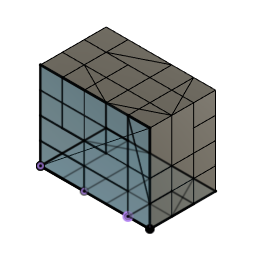
Aula2 v5 (Autodesk Fusion 360 design; units mm, degrees)
Autodesk Fusion 360 part; units mm, degrees
sketch "FRENTE" plane through (0, 0, 0) normal (0, 1, 0) x (1, 0, 0) in component "exercicio1"
  line L0 (0, 0) -> (50, 0)
  line L1 (50, 0) -> (50, -40)
  line L2 (50, -40) -> (0, -40)
  line L3 (0, -40) -> (0, 0)
  line L4 (0, 0) -> (20, 0)
  line L5 (20, 0) -> (20, -10)
  line L6 (20, -10) -> (0, -10)
  line L7 (0, -10) -> (0, 0)
  line L8 (0, -40) -> (30, -40)
  line L9 (30, -40) -> (30, -20)
  line L10 (30, -20) -> (0, -20)
  line L11 (0, -20) -> (0, -40)
  line L12 (50, -40) -> (40, -40)
  line L13 (40, -40) -> (40, 0)
  line L14 (40, 0) -> (50, 0)
  line L15 (50, 0) -> (50, -40)
  dimension "d1" = 50
  dimension "d2" = 40
  dimension "d3" = 10
  dimension "d4" = 10
  dimension "d5" = 20
  dimension "d6" = 20
  dimension "d7" = 30
  constraint horizontal L0
  constraint vertical L1
  constraint horizontal L2
  constraint vertical L3
  constraint coincident L0.start L3.end
  constraint horizontal L4
  constraint vertical L5
  constraint horizontal L6
  constraint vertical L7
  constraint horizontal L8
  constraint vertical L9
  constraint horizontal L10
  constraint vertical L11
  constraint horizontal L12
  constraint vertical L13
  constraint horizontal L14
  constraint vertical L15
  constraint coincident L0 L13.end
  measures "d1" distance of L1.end L2.end
  measures "d2" distance of L0.end L1.end
  measures "d3" distance of L1 L13
  measures "d4" distance of L4.end L5.end
  measures "d5" distance of L5.end L6.end
  measures "d6" distance of L8.end L9.end
  measures "d7" distance of L9.end L10.end
sketch "TOPO" plane through (0, 0, 0) normal (0, 0, 1) x (1, 0, 0) in component "exercicio1"
  line L0 (0, 0) -> (50, 0)
  line L1 (50, 0) -> (50, 30)
  line L2 (50, 30) -> (0, 30)
  line L3 (0, 30) -> (0, 0)
  line L4 (40, 10) -> (50, 10)
  line L5 (50, 10) -> (50, 20)
  line L6 (50, 20) -> (40, 20)
  line L7 (40, 20) -> (40, 10)
  line L8 (0, 0) -> (20, 0)
  line L9 (20, 0) -> (20, 20)
  line L10 (20, 20) -> (0, 20)
  line L11 (0, 20) -> (0, 0)
  point P0 (50, 0)
  point P1 (40, 0)
  point P2 (40, 0)
  point P3 (20, 0)
  dimension "d15" = 30
  constraint horizontal L0
  constraint vertical L1
  constraint horizontal L2
  constraint vertical L3
  constraint coincident L0.start L3.end
  constraint coincident P0 L0.end
  constraint horizontal L4
  constraint vertical L5
  constraint horizontal L6
  constraint vertical L7
  constraint midpoint L1 L5
  constraint coincident L7 P2
  constraint equal L4 L7
  constraint horizontal L8
  constraint vertical L9
  constraint horizontal L10
  constraint vertical L11
  constraint coincident L9 P3
  constraint equal L9 L10
  measures "d15" distance of P0 L1.end
extrude "Extrude1" add sketch "FRENTE" along normal up to surface (30 mm away) contours L0 L3 L4 L5 L6 L7 | L0 L2 L3 L5 L6 L9 L10 L13 | L0 L1 L2 L12 L13 L14 L15 makes body 1 in component "exercicio1"
extrude "Extrude3" cut sketch "TOPO" along normal up to surface (10 mm away) contours L0 L3 L8 L9 L10 L11 bodies 1 in component "exercicio1"
extrude "Extrude4" cut sketch "FRENTE" along normal up to surface (10 mm away) from surface at 10 contours L0 L1 L2 L12 L13 L14 L15 bodies 1 in component "exercicio1"
sketch "Sketch1" plane through (0, 0, 0) normal (0, 1, 0) x (1, 0, 0) in component "Exercicio2"
  line L0 (0, 0) -> (50, 0)
  line L1 (50, 0) -> (50, -40)
  line L2 (50, -40) -> (0, -40)
  line L3 (0, -40) -> (0, 0)
  line L4 (10, -40) -> (30, -40)
  line L5 (30, -40) -> (30, -20)
  line L6 (30, -20) -> (10, -20)
  line L7 (10, -20) -> (10, -40)
  line L8 (40, -40) -> (50, -10)
  dimension "d25" = 40
  dimension "d26" = 20
  dimension "d27" = 20
  dimension "d28" = 50
  dimension "d29" = 10
  dimension "d30" = 10
  dimension "d32" = 10
  constraint horizontal L0
  constraint vertical L1
  constraint horizontal L2
  constraint vertical L3
  constraint coincident L0.start L3.end
  constraint horizontal L4
  constraint vertical L5
  constraint horizontal L6
  constraint vertical L7
  constraint coincident L2 L4.start
  constraint coincident L2 L8.start
  constraint coincident L1 L8.end
  measures "d25" distance of L0.start L2.end
  measures "d26" distance of L5.end L6.end
  measures "d27" distance of L4.end L5.end
  measures "d28" distance of L0.start L0.end
  measures "d29" distance of L0.end L8.end
  measures "d30" distance of L1.end L8.start
  measures "d32" distance of L3 L7
sketch "Sketch2" plane through (0, 0, 0) normal (0, 0, 1) x (1, 0, 0) in component "Exercicio2"
  line L0 (0, 0) -> (50, 0)
  line L1 (50, 0) -> (50, 30)
  line L2 (50, 30) -> (0, 30)
  line L3 (0, 30) -> (0, 0)
  line L4 (0, 0) -> (10, 0)
  line L5 (10, 0) -> (10, 30)
  line L6 (10, 30) -> (0, 30)
  line L7 (0, 30) -> (0, 0)
  line L8 (30, 0) -> (50, 0)
  line L9 (50, 0) -> (50, 30)
  line L10 (50, 30) -> (30, 30)
  line L11 (30, 30) -> (30, 0)
  line L12 (50, 0) -> (40, 0)
  line L13 (40, 0) -> (40, 20)
  line L14 (40, 20) -> (50, 20)
  line L15 (50, 20) -> (50, 0)
  point P0 (50, 0)
  dimension "d33" = 30
  dimension "d34" = 10
  dimension "d35" = 10
  dimension "d36" = 10
  dimension "d37" = 10
  constraint horizontal L0
  constraint vertical L1
  constraint horizontal L2
  constraint vertical L3
  constraint coincident L0.start L3.end
  constraint horizontal L4
  constraint vertical L5
  constraint horizontal L6
  constraint vertical L7
  constraint coincident L2 L5.end
  constraint horizontal L8
  constraint vertical L9
  constraint horizontal L10
  constraint vertical L11
  constraint coincident L0 L8.start
  constraint horizontal L12
  constraint vertical L13
  constraint horizontal L14
  constraint vertical L15
  constraint coincident L15 P0
  measures "d33" distance of L1.end P0
  measures "d34" distance of L10 L14
  measures "d35" distance of L11 L13
  measures "d36" distance of L3 L5
  measures "d37" distance of L1 L13
extrude "Extrude1'" add sketch "Sketch1" along normal up to surface (30 mm away) separate body contours L0 L1 L2 L3 L5 L6 L7 L8 | L1 L2 L8 makes body 2 in component "Exercicio2"
extrude "Extrude2" cut sketch "Sketch1" along normal up to surface (20 mm away) contours L1 L2 L8 bodies 2 in component "Exercicio2"
sketch "Sketch1 (2)" plane through (0, 0, 0) normal (0, 1, 0) x (1, 0, 0) in component "Exercicio3"
  line L0 (0, 0) -> (50, 0)
  line L1 (50, 0) -> (50, -40)
  line L2 (50, -40) -> (0, -40)
  line L3 (0, -40) -> (0, 0)
  line L4 (10, -40) -> (30, -40)
  line L5 (30, -40) -> (30, -20)
  line L6 (30, -20) -> (10, -20)
  line L7 (10, -20) -> (10, -40)
  line L8 (40, -40) -> (50, -10)
  dimension "d42" = 40
  dimension "d43" = 50
  dimension "d44" = 10
  dimension "d45" = 10
  dimension "d46" = 20
  dimension "d48" = 10
  constraint horizontal L0
  constraint vertical L1
  constraint horizontal L2
  constraint vertical L3
  constraint coincident L0.start L3.end
  constraint horizontal L4
  constraint vertical L5
  constraint horizontal L6
  constraint vertical L7
  constraint coincident L2 L4.start
  constraint coincident L2 L8.start
  constraint coincident L1 L8.end
  constraint equal L5 L6
  measures "d42" distance of L0.start L2.end
  measures "d43" distance of L0.start L0.end
  measures "d44" distance of L0.end L8.end
  measures "d45" distance of L1.end L8.start
  measures "d46" distance of L5.end L6.end
  measures "d48" distance of L3 L7
sketch "Sketch2 (2)" plane through (0, 0, 0) normal (0, 0, 1) x (1, 0, 0) in component "Exercicio3"
  line L0 (0, 0) -> (50, 0)
  line L1 (50, 0) -> (50, 30)
  line L2 (50, 30) -> (0, 30)
  line L3 (0, 30) -> (0, 0)
  line L4 (10, 0) -> (30, 0)
  line L5 (30, 0) -> (30, 20)
  line L6 (30, 20) -> (10, 20)
  line L7 (10, 20) -> (10, 0)
  line L8 (40, 30) -> (50, 30)
  line L9 (50, 30) -> (50, 10)
  line L10 (50, 10) -> (40, 10)
  line L11 (40, 10) -> (40, 30)
  point P0 (50, 0)
  point P1 (40, 0)
  dimension "d49" = 20
  dimension "d50" = 30
  dimension "d51" = 20
  dimension "d52" = 10
  dimension "d53" = 20
  constraint horizontal L0
  constraint vertical L1
  constraint horizontal L2
  constraint vertical L3
  constraint coincident L0.start L3.end
  constraint horizontal L4
  constraint vertical L5
  constraint horizontal L6
  constraint vertical L7
  constraint coincident L0 L4.start
  constraint horizontal L8
  constraint vertical L9
  constraint horizontal L10
  constraint vertical L11
  constraint coincident L1 L9.end
  constraint coincident L2 L8.start
  constraint coincident L1 P0
  constraint coincident L11 P1
  measures "d49" distance of L8.start L10.end
  measures "d50" distance of P0 L1.end
  measures "d51" distance of L4.end L5.end
  measures "d52" distance of L3 L7
  measures "d53" distance of L5.end L6.end
extrude "Extrude1''" add sketch "Sketch1 (2)" along normal up to surface (30 mm away) separate body makes body 3 in component "Exercicio3"
extrude "Extrude2'" cut sketch "Sketch1 (2)" along normal up to surface (20 mm away) from surface at 10 contours L1 L2 L8 bodies 3 in component "Exercicio3"
extrude "Extrude3'" cut sketch "Sketch1 (2)" along normal up to surface (20 mm away) contours L2 L4 L5 L6 L7 bodies 3 in component "Exercicio3"
sketch "Sketch1 (3)" plane through (0, 0, 0) normal (0, 1, 0) x (1, 0, 0) in component "Exercicio 4"
  line L0 (0, 0) -> (50, 0)
  line L1 (50, 0) -> (50, -40)
  line L2 (50, -40) -> (0, -40)
  line L3 (0, -40) -> (0, 0)
  line L4 (0, -30) -> (40, -30)
  line L5 (40, -30) -> (40, -10)
  line L6 (40, -10) -> (0, -10)
  line L7 (0, -10) -> (0, -30)
  line L8 (0, 0) -> (20, 0)
  line L9 (20, 0) -> (20, -20)
  line L10 (20, -20) -> (0, -20)
  line L11 (0, -20) -> (0, 0)
  line L12 (50, -40) -> (40, -40)
  line L13 (40, -40) -> (40, -20)
  line L14 (40, -20) -> (50, -20)
  line L15 (50, -20) -> (50, -40)
  dimension "d61" = 50
  dimension "d62" = 40
  dimension "d63" = 20
  dimension "d64" = 20
  dimension "d65" = 20
  dimension "d66" = 40
  dimension "d67" = 10
  dimension "d68" = 20
  constraint horizontal L0
  constraint vertical L1
  constraint horizontal L2
  constraint vertical L3
  constraint coincident L0.start L3.end
  constraint horizontal L4
  constraint vertical L5
  constraint horizontal L6
  constraint vertical L7
  constraint horizontal L8
  constraint vertical L9
  constraint horizontal L10
  constraint vertical L11
  constraint horizontal L12
  constraint vertical L13
  constraint horizontal L14
  constraint vertical L15
  constraint midpoint L3 L7
  measures "d61" distance of L1.end L2.end
  measures "d62" distance of L0.start L2.end
  measures "d63" distance of L4.end L5.end
  measures "d64" distance of L8.end L9.end
  measures "d65" distance of L9.end L10.end
  measures "d66" distance of L4.start L4.end
  measures "d67" distance of L13.end L14.end
  measures "d68" distance of L12.end L13.end
sketch "Sketch2 (3)" plane through (0, 0, 0) normal (0, 0, 1) x (1, 0, 0) in component "Exercicio 4"
  line L0 (0, 0) -> (50, 0)
  line L1 (50, 0) -> (50, 30)
  line L2 (50, 30) -> (0, 30)
  line L3 (0, 30) -> (0, 0)
  line L4 (0, 20) -> (20, 30)
  line L5 (0, 10) -> (40, 10)
  line L6 (40, 10) -> (40, 0)
  line L7 (40, 0) -> (0, 0)
  line L8 (0, 0) -> (0, 10)
  line L9 (40, 30) -> (50, 10)
  point P0 (50, 0)
  dimension "d69" = 30
  dimension "d70" = 10
  dimension "d71" = 10
  dimension "d72" = 20
  dimension "d73" = 10
  dimension "d74" = 40
  dimension "d75" = 10
  constraint horizontal L0
  constraint vertical L1
  constraint horizontal L2
  constraint vertical L3
  constraint coincident L0.start L3.end
  constraint coincident P0 L0.end
  constraint coincident L3 L4.start
  constraint coincident L2 L4.end
  constraint horizontal L5
  constraint vertical L6
  constraint horizontal L7
  constraint vertical L8
  constraint coincident L0 L6.end
  constraint coincident L3 L5.start
  constraint coincident L2 L9.start
  constraint coincident L1 L9.end
  measures "d69" distance of P0 L1.end
  measures "d70" distance of P0 L9.end
  measures "d71" horizontal distance of L9.start L9.end
  measures "d72" horizontal distance of L4.start L4.end
  measures "d73" vertical distance of L4.start L4.end
  measures "d74" distance of L5.start L5.end
  measures "d75" distance of L5.end L6.end
extrude "Extrude1'''" add sketch "Sketch1 (3)" along normal up to surface (30 mm away) separate body makes body 4 in component "Exercicio 4"
extrude "Extrude2''" cut sketch "Sketch1 (3)" along normal up to surface (10 mm away) contours L3 L6 L7 L9 L10 L11 | L3 L4 L5 L6 L7 L9 L10 L13 bodies 4 in component "Exercicio 4"
extrude "Extrude3''" cut sketch "Sketch2 (3)" along normal up to surface (20 mm away) from surface at 20 contours L1 L2 L9 bodies 4 in component "Exercicio 4"
extrude "Extrude4'" cut sketch "Sketch2 (3)" along normal up to surface (20 mm away) contours L2 L3 L4 bodies 4 in component "Exercicio 4"
sketch "Sketch1 (4)" plane through (0, 0, 0) normal (0, 1, 0) x (1, 0, 0) in component "Exercicio 5"
  line L0 (0, 0) -> (50, 0)
  line L1 (50, 0) -> (50, -40)
  line L2 (50, -40) -> (0, -40)
  line L3 (0, -40) -> (0, 0)
  line L4 (0, -10) -> (20, -10)
  line L5 (20, -10) -> (20, -40)
  line L6 (40, -40) -> (40, -20)
  line L7 (40, -20) -> (50, -20)
  line L8 (0, -20) -> (20, -40)
  dimension "d85" = 50
  dimension "d86" = 40
  dimension "d87" = 30
  dimension "d88" = 20
  dimension "d89" = 20
  dimension "d90" = 10
  dimension "d91" = 20
  constraint horizontal L0
  constraint vertical L1
  constraint horizontal L2
  constraint vertical L3
  constraint coincident L0.start L3.end
  constraint coincident L3 L4.start
  constraint perpendicular L3 L4
  constraint coincident L2 L5.end
  constraint perpendicular L2 L5
  constraint coincident L2 L6.start
  constraint perpendicular L2 L6
  constraint coincident L1 L7.end
  constraint perpendicular L1 L7
  constraint coincident L3 L8.start
  measures "d85" distance of L1.end L2.end
  measures "d86" distance of L0.start L2.end
  measures "d87" distance of L4.end L5.end
  measures "d88" vertical distance of L5.end L8.start
  measures "d89" horizontal distance of L5.end L8.start
  measures "d90" distance of L6.end L7.end
  measures "d91" distance of L6.start L6.end
sketch "Sketch2 (4)" plane through (0, 0, 0) normal (0, 0, 1) x (1, 0, 0) in component "Exercicio 5"
  line L0 (0, 0) -> (50, 0)
  line L1 (50, 0) -> (50, 30)
  line L2 (50, 30) -> (0, 30)
  line L3 (0, 30) -> (0, 0)
  line L4 (50, 30) -> (40, 30)
  line L5 (40, 30) -> (40, 20)
  line L6 (40, 20) -> (50, 20)
  line L7 (50, 20) -> (50, 30)
  line L8 (50, 0) -> (40, 0)
  line L9 (40, 0) -> (40, 10)
  line L10 (40, 10) -> (50, 10)
  line L11 (50, 10) -> (50, 0)
  line L12 (0, 0) -> (20, 0)
  line L13 (20, 0) -> (20, 20)
  line L14 (20, 20) -> (0, 20)
  line L15 (0, 20) -> (0, 0)
  line L16 (20, 10) -> (0, 10)
  point P0 (20, 0)
  point P1 (50, 0)
  point P2 (40, 0)
  dimension "d92" = 20
  dimension "d93" = 30
  dimension "d94" = 10
  dimension "d95" = 10
  constraint horizontal L0
  constraint vertical L1
  constraint horizontal L2
  constraint vertical L3
  constraint coincident L0.start L3.end
  constraint horizontal L4
  constraint vertical L5
  constraint horizontal L6
  constraint vertical L7
  constraint horizontal L8
  constraint vertical L9
  constraint horizontal L10
  constraint vertical L11
  constraint horizontal L12
  constraint vertical L13
  constraint horizontal L14
  constraint vertical L15
  constraint midpoint L13 L16.start
  constraint midpoint L15 L16.end
  constraint coincident L13 P0
  constraint coincident P1 L0.end
  constraint collinear L5 L9
  constraint coincident L9 P2
  measures "d92" distance of P0 L13.end
  measures "d93" distance of P1 L1.end
  measures "d94" distance of L4.end L5.end
  measures "d95" distance of P2 L9.end
extrude "Extrude1''''" add sketch "Sketch1 (4)" along normal up to surface (30 mm away) separate body makes body 5 in component "Exercicio 5"
extrude "Extrude2'''" cut sketch "Sketch1 (4)" along normal up to surface (10 mm away) contours L1 L2 L6 L7 bodies 5 in component "Exercicio 5"
extrude "Extrude3'''" cut 1 faces at (43.3333, 10, 26.6667) along direction (0, 1, 0) up to surface (10 mm away) from surface at 10 on bodies 5 bodies 5 in component "Exercicio 5"
extrude "Extrude4''" cut sketch "Sketch1 (4)" along normal up to surface (10 mm away) contours L3 L4 L5 L8 | L2 L3 L8 bodies 5 in component "Exercicio 5"
extrude "Extrude5" cut sketch "Sketch1 (4)" along normal up to surface (20 mm away) contours L2 L3 L8 bodies 5 in component "Exercicio 5"
sketch "Sketch1 (5)" plane through (0, 0, 0) normal (0, 1, 0) x (1, 0, 0) in component "Exercicio 6"
  line L0 (0, 0) -> (50, 0)
  line L1 (50, 0) -> (50, -40)
  line L2 (50, -40) -> (0, -40)
  line L3 (0, -40) -> (0, 0)
  line L4 (0, -40) -> (20, -40)
  line L5 (20, -40) -> (20, -10)
  line L6 (20, -10) -> (0, -10)
  line L7 (0, -10) -> (0, -40)
  line L8 (50, -40) -> (30, -40)
  line L9 (30, -40) -> (30, -20)
  line L10 (30, -20) -> (50, -20)
  line L11 (50, -20) -> (50, -40)
  line L12 (30, -30) -> (50, -30) construction
  dimension "d107" = 40
  dimension "d108" = 30
  dimension "d109" = 20
  dimension "d110" = 20
  dimension "d111" = 20
  dimension "d112" = 50
  constraint horizontal L0
  constraint vertical L1
  constraint horizontal L2
  constraint vertical L3
  constraint coincident L0.start L3.end
  constraint horizontal L4
  constraint vertical L5
  constraint horizontal L6
  constraint vertical L7
  constraint horizontal L8
  constraint vertical L9
  constraint horizontal L10
  constraint vertical L11
  constraint midpoint L9 L12.start
  constraint midpoint L11 L12.end
  measures "d107" distance of L0.start L2.end
  measures "d108" distance of L4.end L5.end
  measures "d109" distance of L5.end L6.end
  measures "d110" distance of L9.end L10.end
  measures "d111" distance of L8.end L9.end
  measures "d112" distance of L0.start L0.end
sketch "Sketch2 (5)" plane through (0, 0, 0) normal (0, 0, 1) x (1, 0, 0) in component "Exercicio 6"
  line L0 (0, 0) -> (50, 0)
  line L1 (50, 0) -> (50, 30)
  line L2 (50, 30) -> (0, 30)
  line L3 (0, 30) -> (0, 0)
  line L4 (0, 0) -> (20, 0)
  line L5 (20, 0) -> (20, 20)
  line L6 (20, 20) -> (0, 20)
  line L7 (0, 20) -> (0, 0)
  line L8 (50, 30) -> (30, 30)
  line L9 (30, 30) -> (30, 20)
  line L10 (30, 20) -> (50, 20)
  line L11 (50, 20) -> (50, 30)
  line L12 (30, 0) -> (50, 10)
  point P0 (50, 0)
  point P1 (30, 0)
  point P2 (20, 0)
  dimension "d113" = 30
  dimension "d114" = 10
  dimension "d115" = 10
  dimension "d116" = 20
  constraint horizontal L0
  constraint vertical L1
  constraint horizontal L2
  constraint vertical L3
  constraint coincident L0.start L3.end
  constraint horizontal L4
  constraint vertical L5
  constraint horizontal L6
  constraint vertical L7
  constraint horizontal L8
  constraint vertical L9
  constraint horizontal L10
  constraint vertical L11
  constraint coincident L0 P1
  constraint coincident L1 L12.end
  constraint coincident P0 L0.end
  constraint coincident P1 L12.start
  constraint coincident L9 P1
  constraint coincident L5 P2
  measures "d113" distance of P0 L1.end
  measures "d114" vertical distance of P1 L12.end
  measures "d115" distance of L2 L10
  measures "d116" distance of P2 L5.end
extrude "Extrude1'''''" add sketch "Sketch2 (5)" along normal up to surface (40 mm away) separate body makes body 6 in component "Exercicio 6"
extrude "Extrude2''''" cut sketch "Sketch2 (5)" along normal up to surface (20 mm away) from surface at 20 contours L0 L1 L12 bodies 6 in component "Exercicio 6"
extrude "Extrude3''''" cut sketch "Sketch2 (5)" along normal up to surface (10 mm away) from surface at 30 contours L1 L2 L8 L9 L10 L11 bodies 6 in component "Exercicio 6"
extrude "Extrude4'''" cut sketch "Sketch1 (5)" along normal up to surface (20 mm away) contours L2 L3 L4 L5 L6 L7 bodies 6 in component "Exercicio 6"
sketch "Sketch1 (6)" plane through (0, 0, 0) normal (0, 1, 0) x (1, 0, 0) in component "Exercicio 7"
  line L0 (0, 0) -> (50, 0)
  line L1 (50, 0) -> (50, -40)
  line L2 (50, -40) -> (0, -40)
  line L3 (0, -40) -> (0, 0)
  line L4 (0, -30) -> (10, -30)
  line L5 (10, -30) -> (10, -10)
  line L6 (10, -10) -> (0, -10)
  line L7 (0, -10) -> (0, -30)
  line L8 (30, -40) -> (30, 0)
  line L9 (40, -40) -> (50, -10)
  dimension "d127" = 40
  dimension "d128" = 50
  dimension "d129" = 10
  dimension "d130" = 30
  dimension "d131" = 20
  dimension "d132" = 10
  dimension "d133" = 20
  constraint horizontal L0
  constraint vertical L1
  constraint horizontal L2
  constraint vertical L3
  constraint coincident L0.start L3.end
  constraint horizontal L4
  constraint vertical L5
  constraint horizontal L6
  constraint vertical L7
  constraint coincident L3 L4.start
  constraint coincident L2 L8.start
  constraint coincident L0 L8.end
  constraint perpendicular L0 L8
  constraint coincident L2 L9.start
  constraint coincident L1 L9.end
  constraint midpoint L3 L7
  measures "d127" distance of L0.start L2.end
  measures "d128" distance of L1.end L2.end
  measures "d129" horizontal distance of L9.start L9.end
  measures "d130" vertical distance of L9.start L9.end
  measures "d131" distance of L1 L8
  measures "d132" distance of L5.end L6.end
  measures "d133" distance of L4.end L5.end
sketch "Sketch2 (6)" plane through (0, 0, 0) normal (0, 0, 1) x (1, 0, 0) in component "Exercicio 7"
  line L0 (0, 0) -> (50, 0)
  line L1 (50, 0) -> (50, 30)
  line L2 (50, 30) -> (0, 30)
  line L3 (0, 30) -> (0, 0)
  line L4 (0, 10) -> (30, 10)
  line L5 (30, 10) -> (30, 20)
  line L6 (30, 20) -> (0, 20)
  line L7 (0, 20) -> (0, 10)
  line L8 (10, 10) -> (10, 20)
  line L9 (50, 30) -> (40, 30)
  line L10 (40, 30) -> (40, 10)
  line L11 (40, 10) -> (50, 10)
  line L12 (50, 10) -> (50, 30)
  line L13 (50, 0) -> (0, 0)
  point P0 (50, 0)
  point P1 (30, 0)
  point P2 (10, 0)
  point P3 (40, 0)
  dimension "d134" = 30
  dimension "d135" = 10
  dimension "d150" = 20
  constraint horizontal L0
  constraint vertical L1
  constraint horizontal L2
  constraint vertical L3
  constraint coincident L0.start L3.end
  constraint horizontal L4
  constraint vertical L5
  constraint horizontal L6
  constraint vertical L7
  constraint coincident L4 L8.start
  constraint coincident L6 L8.end
  constraint perpendicular L6 L8
  constraint midpoint L3 L7
  constraint coincident L1 P0
  constraint coincident L5 P1
  constraint coincident L8 P2
  constraint horizontal L9
  constraint vertical L10
  constraint horizontal L11
  constraint vertical L12
  constraint coincident L10 P3
  measures "d134" distance of P0 L1.end
  measures "d135" distance of L4.end L5.end
  measures "d150" distance of L9.end L10.end
extrude "Extrude1''''''" add sketch "Sketch2 (6)" along normal up to surface (40 mm away) separate body makes body 7 in component "Exercicio 7"
extrude "Extrude6" cut sketch "Sketch1 (6)" along normal up to surface (10 mm away) from surface at 10 contours L0 L2 L3 L4 L5 L6 L8 bodies 7 in component "Exercicio 7"
extrude "Extrude7" cut sketch "Sketch1 (6)" along normal up to surface (20 mm away) from surface at 10 contours L1 L2 L9 bodies 7 in component "Exercicio 7"
sketch "Sketch1 (7)" plane through (0, 0, 0) normal (0, 1, 0) x (1, 0, 0) in component "Exercicio 8"
  line L0 (0, 0) -> (50, 0)
  line L1 (50, 0) -> (50, -40)
  line L2 (50, -40) -> (0, -40)
  line L3 (0, -40) -> (0, 0)
  line L4 (10, -40) -> (30, -40)
  line L5 (30, -40) -> (30, -20)
  line L6 (30, -20) -> (10, -20)
  line L7 (10, -20) -> (10, -40)
  line L8 (30, -40) -> (50, 0)
  dimension "d157" = 40
  dimension "d158" = 50
  dimension "d159" = 20
  dimension "d160" = 20
  dimension "d161" = 10
  constraint horizontal L0
  constraint vertical L1
  constraint horizontal L2
  constraint vertical L3
  constraint coincident L0.start L3.end
  constraint horizontal L4
  constraint vertical L5
  constraint horizontal L6
  constraint vertical L7
  constraint coincident L2 L4.start
  measures "d157" distance of L0.start L2.end
  measures "d158" distance of L1.end L2.end
  measures "d159" distance of L5.end L6.end
  measures "d160" distance of L4.start L6.end
  measures "d161" distance of L3 L7
sketch "Sketch2 (7)" plane through (0, 0, 0) normal (0, 0, 1) x (1, 0, 0) in component "Exercicio 8"
  line L0 (0, 0) -> (50, 0)
  line L1 (50, 0) -> (50, 30)
  line L2 (50, 30) -> (0, 30)
  line L3 (0, 30) -> (0, 0)
  line L4 (50, 20) -> (30, 20)
  line L5 (30, 20) -> (30, 10)
  line L6 (30, 10) -> (50, 10)
  line L7 (50, 10) -> (50, 20)
  line L8 (30, 0) -> (50, 0)
  line L9 (10, 0) -> (10, 10)
  line L10 (10, 10) -> (30, 0)
  line L11 (0, 15) -> (24.9364, 15) construction
  line L12 (10, 30) -> (10, 20)
  line L13 (10, 20) -> (30, 30)
  point P0 (50, 0)
  point P1 (30, 0)
  point P2 (10, 0)
  point P3 (30, 0)
  dimension "d162" = 30
  dimension "d163" = 10
  dimension "d166" = 10
  constraint horizontal L0
  constraint vertical L1
  constraint horizontal L2
  constraint vertical L3
  constraint coincident L0.start L3.end
  constraint coincident L1 P0
  constraint horizontal L4
  constraint vertical L5
  constraint horizontal L6
  constraint vertical L7
  constraint midpoint L1 L7
  constraint coincident L5 P3
  constraint coincident L0 P2
  constraint perpendicular L0 L9
  constraint coincident L0 P3
  constraint coincident L9 P2
  constraint coincident P3 P1
  constraint midpoint L3 L11.start
  constraint perpendicular L3 L11
  constraint symmetric P2 L11 L12.start
  constraint symmetric L9.end L11 L12.end
  constraint symmetric P3 L11 L13.end
  measures "d162" distance of P0 L1.end
  measures "d163" distance of L4.end L5.end
  measures "d166" distance of P2 L9.end
extrude "Extrude1'''''''" add sketch "Sketch1 (7)" along normal up to surface (30 mm away) separate body makes body 8 in component "Exercicio 8"
extrude "Extrude2'''''" cut sketch "Sketch2 (7)" along normal up to surface (20 mm away) from surface at 20 contours L0 L9 L10 bodies 8 in component "Exercicio 8"
ref_plane "WorkPlane1" through (25, 15, 20) normal (0, -1, 0) x (-1, 0, 0) in component "Exercicio 8"
mirror "Mirror1" about plane through (25, 15, 20) normal (0, -1, 0) of "Extrude2'''''" in component "Exercicio 8"
extrude "Extrude3'''''" cut sketch "Sketch1 (7)" along normal up to surface (10 mm away) from surface at 10 contours L1 L2 L8 bodies 8 in component "Exercicio 8"
sketch "Sketch1 (8)" plane through (0, 0, 0) normal (0, 1, 0) x (1, 0, 0) in component "Exercicio 9"
  line L0 (0, 0) -> (50, 0)
  line L1 (50, 0) -> (50, -40)
  line L2 (50, -40) -> (0, -40)
  line L3 (0, -40) -> (0, 0)
  line L4 (0, 0) -> (50, -40)
  dimension "d177" = 40
  dimension "d178" = 50
  constraint horizontal L0
  constraint vertical L1
  constraint horizontal L2
  constraint vertical L3
  constraint coincident L0.start L3.end
  measures "d177" distance of L0.start L2.end
  measures "d178" distance of L1.end L2.end
sketch "Sketch2 (8)" plane through (0, 0, 0) normal (0, 0, 1) x (1, 0, 0) in component "Exercicio 9"
  line L0 (0, 0) -> (50, 0)
  line L1 (50, 0) -> (50, 30)
  line L2 (50, 30) -> (0, 30)
  line L3 (0, 30) -> (0, 0)
  line L4 (0, 10) -> (50, 10)
  line L5 (0, 0) -> (50, 0)
  point P0 (50, 0)
  dimension "d179" = 30
  dimension "d180" = 10
  constraint horizontal L0
  constraint vertical L1
  constraint horizontal L2
  constraint vertical L3
  constraint coincident L0.start L3.end
  constraint coincident L1 P0
  constraint coincident L3 L4.start
  constraint coincident L1 L4.end
  constraint perpendicular L1 L4
  measures "d179" distance of P0 L1.end
  measures "d180" distance of L4 L5
extrude "Extrude1''''''''" add sketch "Sketch1 (8)" along normal up to surface (10 mm away) separate body contours L0 L1 L4 makes body 9 in component "Exercicio 9"
extrude "Extrude2''''''" add sketch "Sketch1 (8)" along normal up to surface (20 mm away) from surface at 10 bodies 9 in component "Exercicio 9"
extrude "Extrude3''''''" add sketch "Sketch1 (8)" along normal up to surface (10 mm away) separate body contours L2 L3 L4 makes body 10 in component "Exercicio 9"
extrude "Extrude4''''" add sketch "Sketch1 (8)" along normal up to surface (20 mm away) from surface at 10 bodies 10 in component "Exercicio 9"
component "exercicio1" placed x (1, 0, 0) y (0, 1, 0) z (0, 0, 1) at (0, 0, 0)
component "Exercicio2" placed x (1, 0, 0) y (0, 1, 0) z (0, 0, 1) at (0, 0, 0)
component "Exercicio3" placed x (1, 0, 0) y (0, 1, 0) z (0, 0, 1) at (0, 0, 0)
component "Exercicio 4" placed x (1, 0, 0) y (0, 1, 0) z (0, 0, 1) at (0, 0, 0)
component "Exercicio 5" placed x (1, 0, 0) y (0, 1, 0) z (0, 0, 1) at (0, 0, 0)
component "Exercicio 6" placed x (1, 0, 0) y (0, 1, 0) z (0, 0, 1) at (0, 0, 0)
component "Exercicio 7" placed x (1, 0, 0) y (0, 1, 0) z (0, 0, 1) at (0, 0, 0)
component "Exercicio 8" placed x (1, 0, 0) y (0, 1, 0) z (0, 0, 1) at (0, 0, 0)
component "Exercicio 9" placed x (1, 0, 0) y (0, 1, 0) z (0, 0, 1) at (0, 0, 0)
hidden bodies 10
equation "d35 = d34"
equation "d36 = d35"
equation "d37 = d35"
equation "d45 = d44"
equation "d46 = d45 * 2"
equation "d48 = d45"
equation "d51 = d49"
